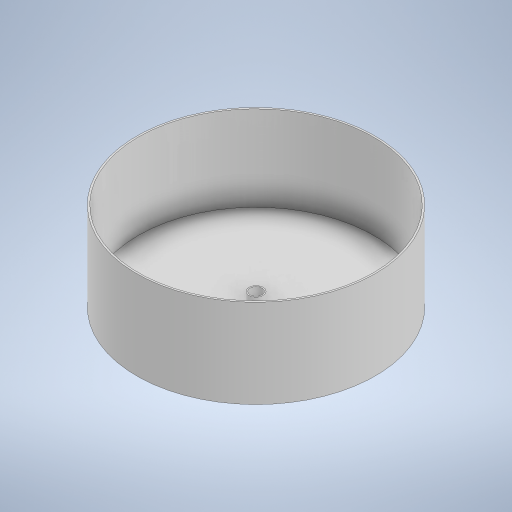
# Autodesk Inventor part: Molde_V002
Saved by Autodesk Inventor 2023 (Build 270158000, 158)
## iProperties
Created: 2022-04-27
Part Number: Molde_V002
Material: Genérico
Document SubType Name: Modeling
Designer: skatl
Density: 1 g/cm^3
Appearance: Valor por defecto
Author: skatl
Autodesk Inventor part; units mm, degrees
ref_plane "YZ Plane" through (0, 0, 0) normal (1, 0, 0) x (0, 1, 0)
ref_plane "XZ Plane" through (0, 0, 0) normal (0, 1, 0) x (-1, 0, 0)
ref_plane "XY Plane" through (0, 0, 0) normal (0, 0, 1) x (1, 0, 0)
sketch "Boceto1" plane through (0, 0, 0) normal (0, 1, 0) x (-1, 0, 0)
  circle A0 centre (0, 0) radius 34.5
  circle A1 centre (0, 0) radius 35
  dimension "d0" = 69
  dimension "d1" = 70
  constraints: 2 centre point, 2 coincident
  measures "d0" diameter of A0
  measures "d1" diameter of A1
extrude "Extrusión1" add sketch "Boceto1" along normal blind 1 contours A0 | A1
sketch "Boceto2" plane through (0, 1, 0) normal (0, 1, 0) x (1, 0, 0)
  circle A0 centre (0, 0) radius 34.5
  circle A1 centre (0, 0) radius 35
  dimension "d4" = 69
  dimension "d5" = 70
  constraints: 2 centre point, 2 coincident
  measures "d4" diameter of A0
  measures "d5" diameter of A1
extrude "Extrusión2" add sketch "Boceto2" along normal blind 25
sketch "Boceto3" plane through (0, 1, 0) normal (0, 1, 0) x (1, 0, 0)
  circle A0 centre (0, 0) radius 2.1
  circle A1 centre (0, 0) radius 1.75
  dimension "d8" = 4.2
  dimension "d9" = 3.5
  constraints: 2 centre point, 2 coincident
  measures "d8" diameter of A0
  measures "d9" diameter of A1
extrude "Extrusión3" add sketch "Boceto3" along normal blind 3
sketch "Boceto4" plane through (0, 1, 0) normal (0, 1, 0) x (1, 0, 0)
  circle A0 centre (0, 0) radius 1.75
  dimension "d14" = 3.5
  constraints: 1 centre point, 1 coincident
  measures "d14" diameter of A0
extrude "Extrusión4" cut sketch "Boceto4" against normal through all
